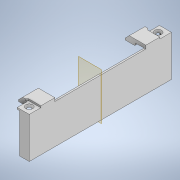
# Autodesk Inventor part: backplate
Saved by Autodesk Inventor 2020.1 (Build 241239000, 239)
## iProperties
Created: 2019-08-16
Part Number: backplate
Material: Generic
Document SubType Name: Modeling
Designer: jjsch
Density: 1 g/cm^3
Appearance: Default
Author: jjsch
Autodesk Inventor part; units mm, degrees
ref_plane "YZ Plane" through (0, 0, 0) normal (1, 0, 0) x (0, 1, 0)
ref_plane "XZ Plane" through (0, 0, 0) normal (0, 1, 0) x (-1, 0, 0)
ref_plane "XY Plane" through (0, 0, 0) normal (0, 0, 1) x (1, 0, 0)
sketch "Sketch1" plane through (0, 0, 0) normal (1, 0, 0) x (0, 1, 0)
  line L0 (0, 0) -> (-47.4, 0)
  line L1 (-47.4, 0) -> (-47.4, 172)
  line L2 (-47.4, 172) -> (0, 172)
  line L3 (0, 172) -> (0, 0)
  dimension "d0" = 172
  dimension "d1" = 47.4
  constraints: 8 end point, 2 parallel, 1 horizontal, 1 perpendicular
  measures "d0" distance of L0.end L1.end
  measures "d1" distance between parallel lines of L3 L1
extrude "Extrusion1" add sketch "Sketch1" along normal blind 2
sketch "Sketch2" plane through (0, 0, 0) normal (-1, 0, 0) x (0, 0, 1)
  line L0 (0, 0) -> (172, 0) projected
  line L1 (172, -47.4) -> (0, -47.4) projected
  line L2 (0, 0) -> (2, 0)
  line L3 (2, 0) -> (2, -47.4)
  line L4 (2, -47.4) -> (0, -47.4)
  line L5 (0, -47.4) -> (0, 0)
  line L6 (172, 0) -> (172, -47.4) projected
  line L7 (0, -47.4) -> (172, -47.4)
  line L8 (172, -47.4) -> (172, -45.4)
  line L9 (172, -45.4) -> (0, -45.4)
  line L10 (0, -45.4) -> (0, -47.4)
  line L11 (172, -47.4) -> (170, -47.4)
  line L12 (170, -47.4) -> (170, 0)
  line L13 (170, 0) -> (172, 0)
  line L14 (172, 0) -> (172, -47.4)
  point P0 (2, -45.4)
  point P1 (0, -47.4)
  point P2 (170, -45.4)
  dimension "d4" = 2
  dimension "d5" = 2
  dimension "d6" = 2
  constraints: 24 end point, 6 parallel, 3 horizontal, 3 perpendicular, 3 point on line
  measures "d4" distance of L3.end L4.end
  measures "d5" distance of L8.end L7.end
  measures "d6" distance of L12.end L13.end
extrude "Extrusion2" add sketch "Sketch2" along normal blind 10 contours L0 L3 L9 L5 | L9 L3 L1 L5 | L0 L6 L9 L12 | L9 L12 L1 L3 | L9 L6 L1 L12
sketch "Sketch3" plane through (2, 0, 172) normal (0, 1, 0) x (1, 0, 0)
  line L0 (0, 0) -> (0, 172) projected
  line L1 (0, 12) -> (-25, 12)
  line L2 (-25, 12) -> (-25, 31)
  line L3 (-25, 31) -> (0, 31)
  line L4 (0, 31) -> (0, 12)
  line L5 (-12, 0) -> (0, 0) projected
  point P0 (-2, 172)
  point P1 (0, 31)
  dimension "d9" = 12
  dimension "d10" = 25
  dimension "d11" = 19
  constraints: 8 end point, 2 parallel, 1 horizontal, 1 perpendicular, 1 point on line
  measures "d9" distance between parallel lines of L5 L1
  measures "d10" distance between parallel lines of L2 L0
  measures "d11" distance of L1.end L2.end
extrude "Extrusion3" add sketch "Sketch3" along normal blind 4
sketch "Sketch4" plane through (2, 0, 172) normal (0, -1, 0) x (1, 0, 0)
  line L0 (-2, -31) -> (-2, -12) projected
  line L1 (0, -12) -> (0, -31) projected
  line L2 (0, -31) -> (-25, -31) projected
  line L3 (-25, -31) -> (-25, -12) projected
  line L4 (-25, -12) -> (0, -12) projected
  line L5 (-25, -31) -> (-25, -12) projected
  line L6 (-2, -31) -> (-25, -31) projected
  line L7 (-25, -12) -> (-12.388, -12)
  line L8 (-12.388, -12) -> (-12.388, -31)
  line L9 (-12.388, -31) -> (-25, -31)
  line L10 (-25, -31) -> (-25, -12)
  point P0 (-2, -172)
  point P1 (-12.388, -12)
  dimension "d14" = 12.388
  constraints: 8 end point, 2 parallel, 1 horizontal, 1 perpendicular, 1 point on line
  measures "d14" distance between parallel lines of L1 L8
extrude "Extrusion4" add sketch "Sketch4" along normal blind 3 contours L2 L3 L4 L8
chamfer "Chamfer1" distance 1 angle 45 1 edges at (-10.388, -3, 150.5)
chamfer "Chamfer2" distance 5 angle 45 1 edges at (-23, 4, 150.5)
sketch "Sketch5" plane through (0, 0, 160) normal (0, 0, 1) x (1, 0, 0)
  line L0 (0, 0) -> (-10, 0) projected
  line L1 (2, 0) -> (-12.5, 0)
  line L2 (-12.5, 0) -> (-12.5, 2)
  line L3 (-12.5, 2) -> (2, 2)
  line L4 (2, 2) -> (2, 0)
  point P0 (-5, 0)
  dimension "d26" = 14.5
  dimension "d27" = 2
  constraints: 8 end point, 2 parallel, 1 horizontal, 1 perpendicular
  measures "d26" distance of L2.end L3.end
  measures "d27" distance of L1.end L2.end
extrude "Extrusion5" add sketch "Sketch5" along normal up to surface (12 mm away)
ref_plane "Work Plane1" through (-10, -47.4, 86) normal (0, 0, 1) x (1, 0, 0)
sketch "Sketch6" plane through (-12.5, 2, 160) normal (0, 1, 0) x (1, 0, 0)
  line L0 (0, -12) -> (14.5, -12) projected
  line L1 (14.5, 0) -> (14.5, -12) projected
  point P0 (12.5, 160)
  point P1 (6.5, -4)
  dimension "d28" = 8
  dimension "d29" = 8
  measures "d28" distance from line of point (6.5, -4) L0
  measures "d29" distance from line of L1 point (6.5, -4)
hole "Hole1" at (-6, 2, 164) direction (0, -1, 0) diameter 4 depth 10 tip angle 118 countersink diameter 8.4 countersink angle 90
sketch "Sketch7" plane through (2, 4, 172) normal (0, 1, 0) x (1, 0, 0)
  line L0 (-20, 12) -> (0, 12) projected
  line L1 (0, 12) -> (-14.5, 12)
  line L2 (-14.5, 12) -> (-14.5, 14)
  line L3 (-14.5, 14) -> (0, 14)
  line L4 (0, 14) -> (0, 12)
  point P0 (-2, 172)
  dimension "d37" = 14.5
  dimension "d38" = 2
  constraints: 8 end point, 2 parallel, 1 horizontal, 1 perpendicular
  measures "d37" distance of L2.end L3.end
  measures "d38" distance of L1.end L2.end
extrude "Extrusion6" cut sketch "Sketch7" against normal up to surface (2 mm away)
chamfer "Chamfer3" distance 2 angle 45 1 edges at (-12.5, 3, 160)
mirror "Mirror2" about plane through (-10, -47.4, 86) normal (0, 0, 1) of "Extrusion3", "Extrusion5", "Hole1", "Chamfer3", "Chamfer2", "Chamfer1", "Extrusion4", "Extrusion6"
sketch "Sketch8" plane through (2, -47.4, 0) normal (0, -1, 0) x (1, 0, 0)
  circle A0 centre (-8, 164) radius 2.2 projected
  circle A1 centre (-8, 164) radius 4.2 projected
  circle A2 centre (-8, 8) radius 4.2 projected
  circle A3 centre (-8, 8) radius 2.2 projected
  circle A4 centre (-8, 8) radius 4.2 projected
  point P0 (-2, 0)
  point P1 (-12, 2)
  constraints: 2 coincident
hole "Hole2" at (-6, -47.4, 8) at (-6, -47.4, 164) direction (0, 1, 0) diameter 4 depth 10 tip angle 118 countersink diameter 8.4 countersink angle 90
body "Solid1"
